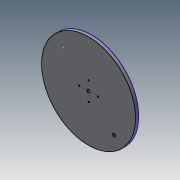
# Autodesk Inventor part: mainpulley
Saved by Autodesk Inventor 2015 (Build 190159000, 159)
## iProperties
Created: 2014-08-31
Part Number: mainpulley
Material: Generic
Document SubType Name: Modeling
Designer: shohei
Density: 1 g/cm^3
Appearance: Default
Mass: 1410.58 g
Surface Area: 1611.64 cm^2
Volume: 1410.58 cm^3
Author: shohei
Autodesk Inventor part; units mm, degrees
ref_plane "YZ Plane" through (0, 0, 0) normal (1, 0, 0) x (0, 1, 0)
ref_plane "XZ Plane" through (0, 0, 0) normal (0, 1, 0) x (-1, 0, 0)
ref_plane "XY Plane" through (0, 0, 0) normal (0, 0, 1) x (1, 0, 0)
sketch "Block1" plane through (0, 0, 0) normal (0, 0, 1) x (1, 0, 0)
  circle A0 centre (0, 0) radius 150.22
  circle A1 centre (0, 0) radius 5.22
  circle A2 centre (-0.0076, 30) radius 2.22
  circle A3 centre (30, 0.0076) radius 2.22
  circle A4 centre (0.0076, -30) radius 2.22
  circle A5 centre (-30, -0.0076) radius 2.22
  circle A6 centre (-81.3173, -81.3173) radius 5.22
  point P0 (-11.6168, -11.6168)
sketch "Sketch1" plane through (0, 0, 0) normal (0, 1, 0) x (-1, 0, 0)
  circle A0 centre (0, 0) radius 150
  circle A1 centre (0, 0) radius 5
  circle A2 centre (81.3173, 81.3173) radius 5
  line L0 (210.308, 0) -> (-210.308, 0) projected
  line L1 (0, -210.308) -> (0, 210.308) projected
  circle A3 centre (0, 10) radius 2
  circle A4 centre (-10, 0) radius 2
  circle A5 centre (0, -10) radius 2
  circle A6 centre (10, 0) radius 2
  dimension "d12" = 360
  dimension "d0" = 300
  dimension "d1" = 10
  dimension "d2" = 10
  dimension "d7" = 105
  dimension "d9" = 4
  dimension "d18" = 10
  constraints: 7 centre point, 3 coincident, 1 point on line, 9 other
  measures "d0" diameter of A0
  measures "d1" diameter of A1
  measures "d2" diameter of A2
  measures "d9" diameter of A3
  measures "d18" distance of A6.centre A1.centre
ref_plane "Work Plane1" through (0, 10, 0) normal (0, 1, 0) x (1, 0, 0)
extrude "Extrusion4" add sketch "Sketch1" along normal blind 10 contours L0 A6 A1 L1 A3 A0 | A0 L1 A5 A1 L0 A6 | L1 A3 A1 L0 A4 A0 | A0 L0 A4 A1 L1 A5
sketch "Sketch4" plane through (0, 0, 0) normal (0, -1, 0) x (1, 0, 0)
  circle A0 centre (-81.3173, 81.3173) radius 5 projected
  circle A1 centre (0, 0) radius 5 projected
  circle A2 centre (-10, 0) radius 2 projected
  circle A3 centre (0, -10) radius 2 projected
  circle A4 centre (10, 0) radius 2 projected
  circle A5 centre (0, 10) radius 2 projected
  circle A6 centre (0, 0) radius 150 projected
  circle A7 centre (0, 0) radius 150.22
  circle A8 centre (-81.3173, 81.3173) radius 5.22
  circle A9 centre (0, 10) radius 2.22
  circle A10 centre (-10, 0) radius 2.22
  circle A11 centre (0, 0) radius 5.22
  circle A12 centre (10, 0) radius 2.22
  circle A13 centre (0, -10) radius 2.22
  dimension "d28" = 0.22
  dimension "d29" = 0.22
  dimension "d30" = 0.22
  dimension "d31" = 0.22
  dimension "d32" = 0.22
  dimension "d33" = 0.22
  dimension "d34" = 0.22
  constraints: 7 centre point
  measures "d28" radial gap between concentric circles of A10 A2
  measures "d29" radial gap between concentric circles of A9 A5
  measures "d30" radial gap between concentric circles of A11 A1
  measures "d31" radial gap between concentric circles of A12 A4
  measures "d32" radial gap between concentric circles of A13 A3
  measures "d33" radial gap between concentric circles of A8 A0
  measures "d34" radial gap between concentric circles of A7 A6
equation "\"d0\" = pD"
equation "\"d7\" = 0.35 * pD"
equation "\"d28\" = Kerf"
equation "\"d29\" = Kerf"
equation "\"d30\" = Kerf"
equation "\"d31\" = Kerf"
equation "\"d32\" = Kerf"
equation "\"d33\" = Kerf"
equation "\"d34\" = Kerf"
equation "\"pD\" = 300"
equation "\"Kerf\" = 0.22"
body "Solid4"
